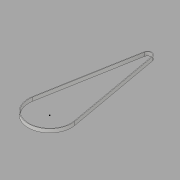
# Autodesk Inventor part: belt_460mm
Saved by Autodesk Inventor 2019 (Build 230136000, 136)
## iProperties
Created: 2021-11-07
Part Number: belt_460mm
Material: Generic
Document SubType Name: Modeling
Designer: Mohamed
Density: 1 g/cm^3
Appearance: Default
Author: Mohamed
Autodesk Inventor part; units mm, degrees
ref_plane "YZ Plane" through (0, 0, 0) normal (1, 0, 0) x (0, 1, 0)
ref_plane "XZ Plane" through (0, 0, 0) normal (0, 1, 0) x (-1, 0, 0)
ref_plane "XY Plane" through (0, 0, 0) normal (0, 0, 1) x (1, 0, 0)
sketch "Sketch1" plane through (0, 0, 0) normal (0, 1, 0) x (-1, 0, 0)
  point P0 (0, 0)
sketch "Sketch2" plane through (0, 0, 0) normal (0, 1, 0) x (-1, 0, 0)
  arc A0 (34.4492, -6.1847) -> (-34.4492, -6.1847) centre (0, 0) ccw
  arc A1 (-6.1516, -163.8044) -> (6.1516, -163.8044) centre (0, -162.7) ccw
  line L0 (34.4492, -6.1847) -> (6.1516, -163.8044)
  line L1 (-34.4492, -6.1847) -> (-6.1516, -163.8044)
  arc A2 (35.4335, -6.3614) -> (-35.4335, -6.3614) centre (0, 0) ccw
  arc A3 (-7.1359, -163.9811) -> (7.1359, -163.9811) centre (0, -162.7) ccw
  line L2 (35.4335, -6.3614) -> (7.1359, -163.9811)
  line L3 (-35.4335, -6.3614) -> (-7.1359, -163.9811)
  dimension "d0" = 70
  dimension "d2" = 12.5
  dimension "d3" = 72
  dimension "d4" = 14.5
  constraints: 8 end point, 8 point on circle, 8 tangent, 4 centre point, 3 coincident
  measures "d0" diameter of A0
  measures "d2" diameter of A1
  measures "d3" diameter of A2
  measures "d4" diameter of A3
extrude "Extrusion1" add sketch "Sketch2" along normal blind 6
body "Solid1"
